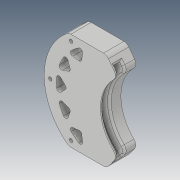
# Autodesk Inventor part: gimbalShroud
Saved by Autodesk Inventor 2018 (Build 220112000, 112)
## iProperties
Created: 2020-01-10
Part Number: gimbalShroud
Material: Generic
Document SubType Name: Modeling
Designer: anirudh
Density: 1 g/cm^3
Appearance: Default
Author: anirudh
Autodesk Inventor part; units mm, degrees
ref_plane "YZ Plane" through (0, 0, 0) normal (1, 0, 0) x (0, 1, 0)
ref_plane "XZ Plane" through (0, 0, 0) normal (0, 1, 0) x (-1, 0, 0)
ref_plane "XY Plane" through (0, 0, 0) normal (0, 0, 1) x (1, 0, 0)
sketch "Sketch1" plane through (0, 0, 0) normal (0, 0, 1) x (1, 0, 0)
  arc A0 (-26.67, 35.56) -> (-26.67, -35.56) centre (0, 0) ccw
  line L0 (-26.67, 35.56) -> (-38.1, 50.8)
  line L1 (-26.67, -35.56) -> (-38.1, -50.8)
  line L2 (-77.47, 50.8) -> (-38.1, 50.8)
  line L3 (-77.47, -50.8) -> (-38.1, -50.8)
  arc A1 (-77.47, 50.8) -> (-77.47, -50.8) centre (-39.37, 0) ccw
  line L4 (-77.47, 50.8) -> (-38.1, 50.8)
  line L5 (-38.1, 50.8) -> (-26.67, 35.56)
  line L6 (-38.1, -50.8) -> (-26.67, -35.56)
  line L7 (-77.47, -50.8) -> (-38.1, -50.8)
  arc A2 (-77.47, 50.8) -> (-77.47, -50.8) centre (-39.37, 0) ccw
  arc A3 (-26.67, 35.56) -> (-26.67, -35.56) centre (0, 0) ccw
  point P0 (-36.5125, 52.3875)
  point P1 (-36.5125, -49.2125)
  constraints: 16 end point, 8 point on circle, 4 centre point, 4 collinear, 2 concentric
extrude "Extrusion1" add sketch "Sketch1" along normal blind 11.938
sketch "Sketch2" plane through (0, 0, 11.938) normal (0, 0, 1) x (1, 0, 0)
  arc A0 (-77.47, 50.8) -> (-77.47, -50.8) centre (-39.37, 0) ccw projected
  arc A1 (-77.47, 50.8) -> (-77.47, -50.8) centre (-39.37, 0) ccw
  arc A2 (-32.385, 43.18) -> (-32.385, -43.18) centre (0, 0) ccw
  line L0 (-38.1, 50.8) -> (-77.47, 50.8) projected
  line L1 (-77.47, 50.8) -> (-38.1, 50.8)
  line L2 (-38.1, 50.8) -> (-32.385, 43.18)
  line L3 (-26.67, 35.56) -> (-38.1, 50.8) projected
  line L4 (-77.47, -50.8) -> (-38.1, -50.8) projected
  line L5 (-77.47, -50.8) -> (-38.1, -50.8)
  line L6 (-38.1, -50.8) -> (-32.385, -43.18)
  line L7 (-38.1, -50.8) -> (-26.67, -35.56) projected
  dimension "d8" = 107.95
  constraints: 8 end point, 4 midpoint, 4 point on circle, 2 centre point, 2 collinear
  measures "d8" diameter of A2
extrude "Extrusion2" add sketch "Sketch2" along normal blind 6.096
sketch "Sketch3" plane through (0, 0, 18.034) normal (0, 0, 1) x (1, 0, 0)
  arc A0 (-77.47, 50.8) -> (-77.47, -50.8) centre (-39.37, 0) ccw projected
  arc A1 (-77.47, 50.8) -> (-77.47, -50.8) centre (-39.37, 0) ccw
  line L0 (-26.67, 35.56) -> (-32.385, 43.18) projected
  arc A2 (-26.67, 35.56) -> (-26.67, -35.56) centre (0, 0) ccw
  line L1 (-38.1, 50.8) -> (-77.47, 50.8) projected
  line L2 (-77.47, 50.8) -> (-38.1, 50.8)
  line L3 (-38.1, 50.8) -> (-26.67, 35.56)
  line L4 (-77.47, -50.8) -> (-38.1, -50.8) projected
  line L5 (-26.67, -35.56) -> (-38.1, -50.8)
  line L6 (-38.1, -50.8) -> (-77.47, -50.8)
  point P0 (0, 0)
  constraints: 8 end point, 4 point on circle, 2 centre point, 1 collinear, 1 horizontal
extrude "Extrusion3" add sketch "Sketch3" along normal blind 3.175
sketch "Sketch4" plane through (0, 0, 21.209) normal (0, 0, 1) x (1, 0, 0)
  arc A0 (-77.47, 50.8) -> (-77.47, -50.8) centre (-39.37, 0) ccw projected
  line L0 (-90.17, 0) -> (-79.0575, 0)
  line L1 (-79.0575, 0) -> (-89.1561, 10.0986)
  line L2 (-79.0575, 0) -> (-64.7759, 0) construction
  line L3 (-79.0575, 0) -> (-89.1561, -10.0986)
  line L4 (-64.1148, -31.0289) -> (-78.3066, -32.628)
  line L5 (-64.1148, -31.0289) -> (-62.5157, -45.2207)
  line L6 (-30.5387, -38.6925) -> (-38.137, -50.785)
  line L7 (-30.5387, -38.6925) -> (-18.4461, -46.2907)
  line L8 (-3.6128, -17.2198) -> (1.1041, -30.6999)
  line L9 (-3.6128, -17.2198) -> (9.8674, -12.5028)
  line L10 (-3.6128, 17.2198) -> (9.8674, 12.5028)
  line L11 (-3.6128, 17.2198) -> (1.1041, 30.6999)
  line L12 (-30.5387, 38.6925) -> (-18.4461, 46.2907)
  line L13 (-30.5387, 38.6925) -> (-38.137, 50.785)
  line L14 (-64.1148, 31.0289) -> (-62.5157, 45.2207)
  line L15 (-64.1148, 31.0289) -> (-78.3066, 32.628)
  arc A1 (-62.5157, 45.2207) -> (-78.3066, 32.628) centre (-39.37, 0) ccw
  arc A2 (-89.1561, 10.0986) -> (-89.1561, -10.0986) centre (-39.37, 0) ccw
  arc A3 (-78.3066, -32.628) -> (-62.5157, -45.2207) centre (-39.37, 0) ccw
  circle A4 centre (-96.52, 0) radius 1.8
  circle A5 centre (-75.0024, -44.6817) radius 1.8
  circle A6 centre (-75.0024, 44.6817) radius 1.8
  arc A7 (-18.4461, 46.2907) -> (-38.137, 50.785) centre (-39.37, 0) ccw
  arc A8 (9.8674, 12.5028) -> (1.1041, 30.6999) centre (-39.37, 0) ccw
  arc A9 (-38.137, -50.785) -> (-18.4461, -46.2907) centre (-39.37, 0) ccw
  arc A10 (1.1041, -30.6999) -> (9.8674, -12.5028) centre (-39.37, 0) ccw
  line L16 (-14.6252, -31.0289) -> (-16.2243, -45.2207)
  line L17 (-14.6252, -31.0289) -> (-0.4334, -32.628)
  line L18 (0.3175, 0) -> (10.4161, -10.0986)
  arc A11 (-16.2243, -45.2207) -> (-0.4334, -32.628) centre (-39.37, 0) ccw
  arc A12 (10.4161, -10.0986) -> (10.4161, 10.0986) centre (-39.37, 0) ccw
  line L19 (0.3175, 0) -> (10.4161, 10.0986)
  line L20 (-14.6252, 31.0289) -> (-0.4334, 32.628)
  line L21 (-14.6252, 31.0289) -> (-16.2243, 45.2207)
  arc A13 (-0.4334, 32.628) -> (-16.2243, 45.2207) centre (-39.37, 0) ccw
  line L22 (-48.2013, 38.6925) -> (-60.2939, 46.2907)
  arc A14 (-40.603, 50.785) -> (-60.2939, 46.2907) centre (-39.37, 0) ccw
  line L23 (-48.2013, 38.6925) -> (-40.603, 50.785)
  line L24 (-75.1272, -17.2198) -> (-88.6074, -12.5028)
  arc A15 (-88.6074, -12.5028) -> (-79.8441, -30.6999) centre (-39.37, 0) ccw
  line L25 (-75.1272, -17.2198) -> (-79.8441, -30.6999)
  line L26 (-85.1392, -22.0413) -> (-75.1272, -17.2198)
  line L27 (-48.2013, -38.6925) -> (-60.2939, -46.2907)
  arc A16 (-60.2939, -46.2907) -> (-40.603, -50.785) centre (-39.37, 0) ccw
  line L28 (-48.2013, -38.6925) -> (-40.603, -50.785)
  line L29 (-75.1272, 17.2198) -> (-88.6074, 12.5028)
  arc A17 (-79.8441, 30.6999) -> (-88.6074, 12.5028) centre (-39.37, 0) ccw
  line L30 (-75.1272, 17.2198) -> (-79.8441, 30.6999)
  line L31 (-3.6128, -17.2198) -> (1.1041, -30.6999)
  line L32 (-3.6128, -17.2198) -> (9.8674, -12.5028)
  line L33 (-3.6128, 17.2198) -> (9.8674, 12.5028)
  arc A18 (1.1041, -30.6999) -> (9.8674, -12.5028) centre (-39.37, 0) ccw
  arc A19 (9.8674, 12.5028) -> (1.1041, 30.6999) centre (-39.37, 0) ccw
  line L34 (-3.6128, 17.2198) -> (1.1041, 30.6999)
  line L35 (-30.5387, 38.6925) -> (-18.4461, 46.2907)
  line L36 (-30.5387, 38.6925) -> (-38.137, 50.785)
  arc A20 (-18.4461, 46.2907) -> (-38.137, 50.785) centre (-39.37, 0) ccw
  line L37 (-64.1148, 31.0289) -> (-78.3066, 32.628)
  arc A21 (-62.5157, 45.2207) -> (-78.3066, 32.628) centre (-39.37, 0) ccw
  line L38 (-64.1148, 31.0289) -> (-62.5157, 45.2207)
  line L39 (-64.1148, -31.0289) -> (-78.3066, -32.628)
  arc A22 (-78.3066, -32.628) -> (-62.5157, -45.2207) centre (-39.37, 0) ccw
  line L40 (-64.1148, -31.0289) -> (-62.5157, -45.2207)
  line L41 (-71.0433, -39.717) -> (-64.1148, -31.0289)
  line L42 (-30.5387, -38.6925) -> (-38.137, -50.785)
  arc A23 (-38.137, -50.785) -> (-18.4461, -46.2907) centre (-39.37, 0) ccw
  line L43 (-30.5387, -38.6925) -> (-18.4461, -46.2907)
  line L44 (-79.0575, 0) -> (-89.1561, -10.0986)
  arc A24 (-89.1561, 10.0986) -> (-89.1561, -10.0986) centre (-39.37, 0) ccw
  line L45 (-79.0575, 0) -> (-89.1561, 10.0986)
  line L46 (0.3175, 0) -> (10.4161, -10.0986)
  line L47 (0.3175, 0) -> (10.4161, 10.0986)
  line L48 (-14.6252, 31.0289) -> (-0.4334, 32.628)
  arc A25 (10.4161, -10.0986) -> (10.4161, 10.0986) centre (-39.37, 0) ccw
  arc A26 (-0.4334, 32.628) -> (-16.2243, 45.2207) centre (-39.37, 0) ccw
  line L49 (-14.6252, 31.0289) -> (-16.2243, 45.2207)
  line L50 (-48.2013, 38.6925) -> (-40.603, 50.785)
  line L51 (-48.2013, 38.6925) -> (-60.2939, 46.2907)
  arc A27 (-40.603, 50.785) -> (-60.2939, 46.2907) centre (-39.37, 0) ccw
  line L52 (-75.1272, 17.2198) -> (-88.6074, 12.5028)
  arc A28 (-79.8441, 30.6999) -> (-88.6074, 12.5028) centre (-39.37, 0) ccw
  line L53 (-75.1272, 17.2198) -> (-79.8441, 30.6999)
  line L54 (-48.2013, -38.6925) -> (-60.2939, -46.2907)
  arc A29 (-60.2939, -46.2907) -> (-40.603, -50.785) centre (-39.37, 0) ccw
  line L55 (-48.2013, -38.6925) -> (-40.603, -50.785)
  line L56 (-50.6741, -49.5263) -> (-48.2013, -38.6925)
  line L57 (-14.6252, -31.0289) -> (-16.2243, -45.2207)
  arc A30 (-16.2243, -45.2207) -> (-0.4334, -32.628) centre (-39.37, 0) ccw
  line L58 (-14.6252, -31.0289) -> (-0.4334, -32.628)
  line L59 (-75.1272, -17.2198) -> (-79.8441, -30.6999)
  arc A31 (-88.6074, -12.5028) -> (-79.8441, -30.6999) centre (-39.37, 0) ccw
  line L60 (-75.1272, -17.2198) -> (-88.6074, -12.5028)
  line L61 (-3.6128, 17.2198) -> (9.8674, 12.5028)
  line L62 (-3.6128, 17.2198) -> (1.1041, 30.6999)
  line L63 (-30.5387, 38.6925) -> (-18.4461, 46.2907)
  arc A32 (9.8674, 12.5028) -> (1.1041, 30.6999) centre (-39.37, 0) ccw
  arc A33 (-18.4461, 46.2907) -> (-38.137, 50.785) centre (-39.37, 0) ccw
  line L64 (-30.5387, 38.6925) -> (-38.137, 50.785)
  line L65 (-64.1148, 31.0289) -> (-62.5157, 45.2207)
  line L66 (-64.1148, 31.0289) -> (-78.3066, 32.628)
  arc A34 (-62.5157, 45.2207) -> (-78.3066, 32.628) centre (-39.37, 0) ccw
  line L67 (-79.0575, 0) -> (-89.1561, -10.0986)
  arc A35 (-89.1561, 10.0986) -> (-89.1561, -10.0986) centre (-39.37, 0) ccw
  line L68 (-79.0575, 0) -> (-89.1561, 10.0986)
  line L69 (-30.5387, -38.6925) -> (-38.137, -50.785)
  arc A36 (-38.137, -50.785) -> (-18.4461, -46.2907) centre (-39.37, 0) ccw
  line L70 (-30.5387, -38.6925) -> (-18.4461, -46.2907)
  line L71 (-28.0659, -49.5263) -> (-30.5387, -38.6925)
  line L72 (-3.6128, -17.2198) -> (1.1041, -30.6999)
  arc A37 (1.1041, -30.6999) -> (9.8674, -12.5028) centre (-39.37, 0) ccw
  line L73 (-3.6128, -17.2198) -> (9.8674, -12.5028)
  line L74 (-64.1148, -31.0289) -> (-62.5157, -45.2207)
  arc A38 (-78.3066, -32.628) -> (-62.5157, -45.2207) centre (-39.37, 0) ccw
  line L75 (-64.1148, -31.0289) -> (-78.3066, -32.628)
  line L76 (-14.6252, 31.0289) -> (-0.4334, 32.628)
  line L77 (-14.6252, 31.0289) -> (-16.2243, 45.2207)
  line L78 (-48.2013, 38.6925) -> (-40.603, 50.785)
  arc A39 (-0.4334, 32.628) -> (-16.2243, 45.2207) centre (-39.37, 0) ccw
  arc A40 (-40.603, 50.785) -> (-60.2939, 46.2907) centre (-39.37, 0) ccw
  line L79 (-48.2013, 38.6925) -> (-60.2939, 46.2907)
  line L80 (-75.1272, 17.2198) -> (-79.8441, 30.6999)
  line L81 (-75.1272, 17.2198) -> (-88.6074, 12.5028)
  arc A41 (-79.8441, 30.6999) -> (-88.6074, 12.5028) centre (-39.37, 0) ccw
  line L82 (-75.1272, -17.2198) -> (-79.8441, -30.6999)
  arc A42 (-88.6074, -12.5028) -> (-79.8441, -30.6999) centre (-39.37, 0) ccw
  line L83 (-75.1272, -17.2198) -> (-88.6074, -12.5028)
  line L84 (-14.6252, -31.0289) -> (-16.2243, -45.2207)
  arc A43 (-16.2243, -45.2207) -> (-0.4334, -32.628) centre (-39.37, 0) ccw
  line L85 (-14.6252, -31.0289) -> (-0.4334, -32.628)
  line L86 (-7.6967, -39.717) -> (-14.6252, -31.0289)
  line L87 (0.3175, 0) -> (10.4161, -10.0986)
  arc A44 (10.4161, -10.0986) -> (10.4161, 10.0986) centre (-39.37, 0) ccw
  line L88 (0.3175, 0) -> (10.4161, 10.0986)
  line L89 (-48.2013, -38.6925) -> (-40.603, -50.785)
  arc A45 (-60.2939, -46.2907) -> (-40.603, -50.785) centre (-39.37, 0) ccw
  line L90 (-48.2013, -38.6925) -> (-60.2939, -46.2907)
  line L91 (-30.5387, 38.6925) -> (-18.4461, 46.2907)
  line L92 (-30.5387, 38.6925) -> (-38.137, 50.785)
  line L93 (-64.1148, 31.0289) -> (-62.5157, 45.2207)
  arc A46 (-18.4461, 46.2907) -> (-38.137, 50.785) centre (-39.37, 0) ccw
  arc A47 (-62.5157, 45.2207) -> (-78.3066, 32.628) centre (-39.37, 0) ccw
  line L94 (-64.1148, 31.0289) -> (-78.3066, 32.628)
  line L95 (-79.0575, 0) -> (-89.1561, 10.0986)
  line L96 (-79.0575, 0) -> (-89.1561, -10.0986)
  arc A48 (-89.1561, 10.0986) -> (-89.1561, -10.0986) centre (-39.37, 0) ccw
  line L97 (-64.1148, -31.0289) -> (-62.5157, -45.2207)
  arc A49 (-78.3066, -32.628) -> (-62.5157, -45.2207) centre (-39.37, 0) ccw
  line L98 (-64.1148, -31.0289) -> (-78.3066, -32.628)
  line L99 (-3.6128, -17.2198) -> (1.1041, -30.6999)
  arc A50 (1.1041, -30.6999) -> (9.8674, -12.5028) centre (-39.37, 0) ccw
  line L100 (-3.6128, -17.2198) -> (9.8674, -12.5028)
  line L101 (6.3992, -22.0413) -> (-3.6128, -17.2198)
  line L102 (-3.6128, 17.2198) -> (9.8674, 12.5028)
  arc A51 (9.8674, 12.5028) -> (1.1041, 30.6999) centre (-39.37, 0) ccw
  line L103 (-3.6128, 17.2198) -> (1.1041, 30.6999)
  line L104 (-30.5387, -38.6925) -> (-18.4461, -46.2907)
  arc A52 (-38.137, -50.785) -> (-18.4461, -46.2907) centre (-39.37, 0) ccw
  line L105 (-30.5387, -38.6925) -> (-38.137, -50.785)
  line L106 (-48.2013, 38.6925) -> (-40.603, 50.785)
  line L107 (-48.2013, 38.6925) -> (-60.2939, 46.2907)
  line L108 (-75.1272, 17.2198) -> (-79.8441, 30.6999)
  arc A53 (-40.603, 50.785) -> (-60.2939, 46.2907) centre (-39.37, 0) ccw
  arc A54 (-79.8441, 30.6999) -> (-88.6074, 12.5028) centre (-39.37, 0) ccw
  line L109 (-75.1272, 17.2198) -> (-88.6074, 12.5028)
  line L110 (-75.1272, -17.2198) -> (-88.6074, -12.5028)
  line L111 (-75.1272, -17.2198) -> (-79.8441, -30.6999)
  arc A55 (-88.6074, -12.5028) -> (-79.8441, -30.6999) centre (-39.37, 0) ccw
  line L112 (-48.2013, -38.6925) -> (-40.603, -50.785)
  arc A56 (-60.2939, -46.2907) -> (-40.603, -50.785) centre (-39.37, 0) ccw
  line L113 (-48.2013, -38.6925) -> (-60.2939, -46.2907)
  line L114 (0.3175, 0) -> (10.4161, -10.0986)
  arc A57 (10.4161, -10.0986) -> (10.4161, 10.0986) centre (-39.37, 0) ccw
  line L115 (0.3175, 0) -> (10.4161, 10.0986)
  line L116 (11.43, 0) -> (0.3175, 0)
  line L117 (-14.6252, 31.0289) -> (-0.4334, 32.628)
  arc A58 (-0.4334, 32.628) -> (-16.2243, 45.2207) centre (-39.37, 0) ccw
  line L118 (-14.6252, 31.0289) -> (-16.2243, 45.2207)
  line L119 (-14.6252, -31.0289) -> (-0.4334, -32.628)
  arc A59 (-16.2243, -45.2207) -> (-0.4334, -32.628) centre (-39.37, 0) ccw
  line L120 (-14.6252, -31.0289) -> (-16.2243, -45.2207)
  line L121 (-64.1148, 31.0289) -> (-62.5157, 45.2207)
  line L122 (-64.1148, 31.0289) -> (-78.3066, 32.628)
  line L123 (-79.0575, 0) -> (-89.1561, 10.0986)
  arc A60 (-62.5157, 45.2207) -> (-78.3066, 32.628) centre (-39.37, 0) ccw
  arc A61 (-89.1561, 10.0986) -> (-89.1561, -10.0986) centre (-39.37, 0) ccw
  line L124 (-79.0575, 0) -> (-89.1561, -10.0986)
  line L125 (-64.1148, -31.0289) -> (-78.3066, -32.628)
  line L126 (-64.1148, -31.0289) -> (-62.5157, -45.2207)
  arc A62 (-78.3066, -32.628) -> (-62.5157, -45.2207) centre (-39.37, 0) ccw
  line L127 (-30.5387, -38.6925) -> (-18.4461, -46.2907)
  arc A63 (-38.137, -50.785) -> (-18.4461, -46.2907) centre (-39.37, 0) ccw
  line L128 (-30.5387, -38.6925) -> (-38.137, -50.785)
  line L129 (-3.6128, 17.2198) -> (9.8674, 12.5028)
  arc A64 (9.8674, 12.5028) -> (1.1041, 30.6999) centre (-39.37, 0) ccw
  line L130 (-3.6128, 17.2198) -> (1.1041, 30.6999)
  line L131 (6.3992, 22.0413) -> (-3.6128, 17.2198)
  line L132 (-30.5387, 38.6925) -> (-18.4461, 46.2907)
  arc A65 (-18.4461, 46.2907) -> (-38.137, 50.785) centre (-39.37, 0) ccw
  line L133 (-30.5387, 38.6925) -> (-38.137, 50.785)
  line L134 (-3.6128, -17.2198) -> (9.8674, -12.5028)
  arc A66 (1.1041, -30.6999) -> (9.8674, -12.5028) centre (-39.37, 0) ccw
  line L135 (-3.6128, -17.2198) -> (1.1041, -30.6999)
  line L136 (-75.1272, 17.2198) -> (-79.8441, 30.6999)
  line L137 (-75.1272, 17.2198) -> (-88.6074, 12.5028)
  line L138 (-75.1272, -17.2198) -> (-88.6074, -12.5028)
  arc A67 (-79.8441, 30.6999) -> (-88.6074, 12.5028) centre (-39.37, 0) ccw
  arc A68 (-88.6074, -12.5028) -> (-79.8441, -30.6999) centre (-39.37, 0) ccw
  line L139 (-75.1272, -17.2198) -> (-79.8441, -30.6999)
  line L140 (-48.2013, -38.6925) -> (-60.2939, -46.2907)
  line L141 (-48.2013, -38.6925) -> (-40.603, -50.785)
  arc A69 (-60.2939, -46.2907) -> (-40.603, -50.785) centre (-39.37, 0) ccw
  line L142 (-14.6252, -31.0289) -> (-0.4334, -32.628)
  arc A70 (-16.2243, -45.2207) -> (-0.4334, -32.628) centre (-39.37, 0) ccw
  line L143 (-14.6252, -31.0289) -> (-16.2243, -45.2207)
  line L144 (-14.6252, 31.0289) -> (-0.4334, 32.628)
  arc A71 (-0.4334, 32.628) -> (-16.2243, 45.2207) centre (-39.37, 0) ccw
  line L145 (-14.6252, 31.0289) -> (-16.2243, 45.2207)
  line L146 (-7.6967, 39.717) -> (-14.6252, 31.0289)
  line L147 (-48.2013, 38.6925) -> (-40.603, 50.785)
  arc A72 (-40.603, 50.785) -> (-60.2939, 46.2907) centre (-39.37, 0) ccw
  line L148 (-48.2013, 38.6925) -> (-60.2939, 46.2907)
  line L149 (0.3175, 0) -> (10.4161, 10.0986)
  arc A73 (10.4161, -10.0986) -> (10.4161, 10.0986) centre (-39.37, 0) ccw
  line L150 (0.3175, 0) -> (10.4161, -10.0986)
  line L151 (-79.0575, 0) -> (-89.1561, 10.0986)
  line L152 (-79.0575, 0) -> (-89.1561, -10.0986)
  line L153 (-64.1148, -31.0289) -> (-78.3066, -32.628)
  arc A74 (-89.1561, 10.0986) -> (-89.1561, -10.0986) centre (-39.37, 0) ccw
  arc A75 (-78.3066, -32.628) -> (-62.5157, -45.2207) centre (-39.37, 0) ccw
  line L154 (-64.1148, -31.0289) -> (-62.5157, -45.2207)
  line L155 (-30.5387, -38.6925) -> (-38.137, -50.785)
  line L156 (-30.5387, -38.6925) -> (-18.4461, -46.2907)
  arc A76 (-38.137, -50.785) -> (-18.4461, -46.2907) centre (-39.37, 0) ccw
  line L157 (-3.6128, -17.2198) -> (9.8674, -12.5028)
  arc A77 (1.1041, -30.6999) -> (9.8674, -12.5028) centre (-39.37, 0) ccw
  line L158 (-3.6128, -17.2198) -> (1.1041, -30.6999)
  line L159 (-30.5387, 38.6925) -> (-18.4461, 46.2907)
  arc A78 (-18.4461, 46.2907) -> (-38.137, 50.785) centre (-39.37, 0) ccw
  line L160 (-30.5387, 38.6925) -> (-38.137, 50.785)
  line L161 (-28.0659, 49.5263) -> (-30.5387, 38.6925)
  line L162 (-64.1148, 31.0289) -> (-62.5157, 45.2207)
  arc A79 (-62.5157, 45.2207) -> (-78.3066, 32.628) centre (-39.37, 0) ccw
  line L163 (-64.1148, 31.0289) -> (-78.3066, 32.628)
  line L164 (-3.6128, 17.2198) -> (1.1041, 30.6999)
  arc A80 (9.8674, 12.5028) -> (1.1041, 30.6999) centre (-39.37, 0) ccw
  line L165 (-3.6128, 17.2198) -> (9.8674, 12.5028)
  line L166 (-75.1272, -17.2198) -> (-88.6074, -12.5028)
  line L167 (-75.1272, -17.2198) -> (-79.8441, -30.6999)
  line L168 (-48.2013, -38.6925) -> (-60.2939, -46.2907)
  arc A81 (-88.6074, -12.5028) -> (-79.8441, -30.6999) centre (-39.37, 0) ccw
  arc A82 (-60.2939, -46.2907) -> (-40.603, -50.785) centre (-39.37, 0) ccw
  line L169 (-48.2013, -38.6925) -> (-40.603, -50.785)
  line L170 (-14.6252, -31.0289) -> (-16.2243, -45.2207)
  line L171 (-14.6252, -31.0289) -> (-0.4334, -32.628)
  arc A83 (-16.2243, -45.2207) -> (-0.4334, -32.628) centre (-39.37, 0) ccw
  line L172 (0.3175, 0) -> (10.4161, 10.0986)
  arc A84 (10.4161, -10.0986) -> (10.4161, 10.0986) centre (-39.37, 0) ccw
  line L173 (0.3175, 0) -> (10.4161, -10.0986)
  line L174 (-48.2013, 38.6925) -> (-40.603, 50.785)
  arc A85 (-40.603, 50.785) -> (-60.2939, 46.2907) centre (-39.37, 0) ccw
  line L175 (-48.2013, 38.6925) -> (-60.2939, 46.2907)
  line L176 (-50.6741, 49.5263) -> (-48.2013, 38.6925)
  line L177 (-75.1272, 17.2198) -> (-79.8441, 30.6999)
  arc A86 (-79.8441, 30.6999) -> (-88.6074, 12.5028) centre (-39.37, 0) ccw
  line L178 (-75.1272, 17.2198) -> (-88.6074, 12.5028)
  line L179 (-14.6252, 31.0289) -> (-16.2243, 45.2207)
  arc A87 (-0.4334, 32.628) -> (-16.2243, 45.2207) centre (-39.37, 0) ccw
  line L180 (-14.6252, 31.0289) -> (-0.4334, 32.628)
  line L181 (-64.1148, -31.0289) -> (-78.3066, -32.628)
  line L182 (-64.1148, -31.0289) -> (-62.5157, -45.2207)
  line L183 (-30.5387, -38.6925) -> (-38.137, -50.785)
  arc A88 (-78.3066, -32.628) -> (-62.5157, -45.2207) centre (-39.37, 0) ccw
  arc A89 (-38.137, -50.785) -> (-18.4461, -46.2907) centre (-39.37, 0) ccw
  line L184 (-30.5387, -38.6925) -> (-18.4461, -46.2907)
  line L185 (-3.6128, -17.2198) -> (1.1041, -30.6999)
  line L186 (-3.6128, -17.2198) -> (9.8674, -12.5028)
  arc A90 (1.1041, -30.6999) -> (9.8674, -12.5028) centre (-39.37, 0) ccw
  line L187 (-3.6128, 17.2198) -> (1.1041, 30.6999)
  arc A91 (9.8674, 12.5028) -> (1.1041, 30.6999) centre (-39.37, 0) ccw
  line L188 (-3.6128, 17.2198) -> (9.8674, 12.5028)
  line L189 (-64.1148, 31.0289) -> (-62.5157, 45.2207)
  arc A92 (-62.5157, 45.2207) -> (-78.3066, 32.628) centre (-39.37, 0) ccw
  line L190 (-64.1148, 31.0289) -> (-78.3066, 32.628)
  line L191 (-71.0433, 39.717) -> (-64.1148, 31.0289)
  line L192 (-79.0575, 0) -> (-89.1561, 10.0986)
  arc A93 (-89.1561, 10.0986) -> (-89.1561, -10.0986) centre (-39.37, 0) ccw
  line L193 (-79.0575, 0) -> (-89.1561, -10.0986)
  line L194 (-30.5387, 38.6925) -> (-38.137, 50.785)
  arc A94 (-18.4461, 46.2907) -> (-38.137, 50.785) centre (-39.37, 0) ccw
  line L195 (-30.5387, 38.6925) -> (-18.4461, 46.2907)
  line L196 (-48.2013, -38.6925) -> (-60.2939, -46.2907)
  line L197 (-48.2013, -38.6925) -> (-40.603, -50.785)
  line L198 (-14.6252, -31.0289) -> (-16.2243, -45.2207)
  arc A95 (-60.2939, -46.2907) -> (-40.603, -50.785) centre (-39.37, 0) ccw
  arc A96 (-16.2243, -45.2207) -> (-0.4334, -32.628) centre (-39.37, 0) ccw
  line L199 (-14.6252, -31.0289) -> (-0.4334, -32.628)
  line L200 (0.3175, 0) -> (10.4161, -10.0986)
  line L201 (0.3175, 0) -> (10.4161, 10.0986)
  arc A97 (10.4161, -10.0986) -> (10.4161, 10.0986) centre (-39.37, 0) ccw
  line L202 (-14.6252, 31.0289) -> (-16.2243, 45.2207)
  arc A98 (-0.4334, 32.628) -> (-16.2243, 45.2207) centre (-39.37, 0) ccw
  line L203 (-14.6252, 31.0289) -> (-0.4334, 32.628)
  line L204 (-75.1272, 17.2198) -> (-79.8441, 30.6999)
  arc A99 (-79.8441, 30.6999) -> (-88.6074, 12.5028) centre (-39.37, 0) ccw
  line L205 (-75.1272, 17.2198) -> (-88.6074, 12.5028)
  line L206 (-85.1392, 22.0413) -> (-75.1272, 17.2198)
  line L207 (-75.1272, -17.2198) -> (-88.6074, -12.5028)
  arc A100 (-88.6074, -12.5028) -> (-79.8441, -30.6999) centre (-39.37, 0) ccw
  line L208 (-75.1272, -17.2198) -> (-79.8441, -30.6999)
  line L209 (-48.2013, 38.6925) -> (-60.2939, 46.2907)
  arc A101 (-40.603, 50.785) -> (-60.2939, 46.2907) centre (-39.37, 0) ccw
  line L210 (-48.2013, 38.6925) -> (-40.603, 50.785)
  point P0 (0, 0)
  dimension "d19" = 360
  dimension "d21" = 3.6
  dimension "d22" = 3.6
  dimension "d23" = 3.6
  dimension "d29" = 360
  constraints: 422 end point, 210 point on circle, 101 centre point, 2 horizontal, 1 equal length, 667 other
  measures "d21" diameter of A4
  measures "d22" diameter of A5
  measures "d23" diameter of A6
fillet "Fillet1" radius 6.35 8 edges at (-77.47, 50.8, 10.6045) (-77.47, -50.8, 10.6045) (-38.1, -50.8, 10.6045) (-38.1, 50.8, 10.6045) (-26.67, 35.56, 19.6215) (-26.67, 35.56, 5.969) (-26.67, -35.56, 19.6215) (-26.67, -35.56, 5.969)
extrude "Extrusion5" cut sketch "Sketch4" against normal blind 25.4 contours A2 L1 L0 | L0 L3 A2 | L41 A3 L4 | L5 A3 L41 | L191 A1 L14 | L15 A1 L191 | A4 | A5 | A6 | L26 A15 L24 | L25 A15 L26 | L206 A17 L30 | L29 A17 L206
fillet "Fillet2" radius 2.54 15 edges at (-78.3066, 32.628, 10.6045) (-64.1148, 31.0289, 10.6045) (-62.5157, 45.2207, 10.6045) (-75.1272, 17.2198, 10.6045) (-88.6074, 12.5028, 10.6045) (-79.8441, 30.6999, 10.6045) (-79.0575, 0, 10.6045) (-89.1561, 10.0986, 10.6045) (-89.1561, -10.0986, 10.6045) (-75.1272, -17.2198, 10.6045) (-79.8441, -30.6999, 10.6045) (-88.6074, -12.5028, 10.6045) (-78.3066, -32.628, 10.6045) (-64.1148, -31.0289, 10.6045) (-62.5157, -45.2207, 10.6045)
chamfer "Chamfer1" distance 1.905 angle 45 12 edges at (-44.45, 0, 18.034) (-28.9909, 36.0086, 18.034) (-31.313, 41.7506, 18.034) (-28.9909, -36.0086, 18.034) (-31.313, -41.7506, 18.034) (-44.45, 0, 11.938) (-28.9909, 36.0086, 11.938) (-31.313, 41.7506, 11.938) (-28.9909, -36.0086, 11.938) (-31.313, -41.7506, 11.938) (-32.385, 43.18, 14.986) (-32.385, -43.18, 14.986)
body "Solid1"
